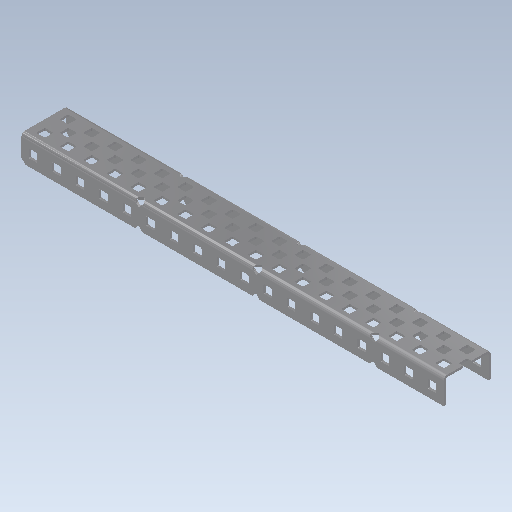
# Autodesk Inventor part: C-Channel 1x3x1x20 hole
Saved by Autodesk Inventor 2020.2 (Build 242310000, 310)
## iProperties
Created: 2012-03-22
Part Number: C-Channel 1x3x1x20 hole
Material: Aluminum 6061
Document SubType Name: Sheet Metal
Designer: Autodesk Inc.
Density: 2.7 g/cm^3
Sheet Metal Rule: Default
Vendor: VEX
Appearance: Aluminum - Polished
Category: Structure
Company: Autodesk Inc.
d52: 0.000 in
d53: 0.000 in
d54: 0.000 in
d55: 0.000 in
d56: 0.000 in
d57: 0.000 in
d58: 0.000 in
d59: 0.000 in
d60: 0.000 in
d61: 0.000 in
d62: 0.000 in
d63: 0.000 in
d64: 0.000 in
d65: 0.000 in
d66: 0.000 in
d67: 0.000 in
d68: 0.000 in
d69: 0.000 in
d70: 0.000 in
d71: 0.000 in
d72: 0.000 in
d73: 0.000 in
d74: 0.000 in
d75: 0.000 in
d76: 0.000 in
d77: 0.000 in
d78: 0.000 in
d79: 0.000 in
d80: 0.000 in
d81: 0.000 in
d82: 0.000 in
d83: 0.000 in
d84: 0.000 in
d85: 0.000 in
d86: 0.000 in
d87: 0.000 in
d88: 0.000 in
d89: 0.000 in
d90: 0.000 in
d91: 0.000 in
d92: 0.000 in
d93: 0.000 in
d94: 0.000 in
d95: 0.000 in
d96: 0.000 in
d97: 0.000 in
d98: 0.000 in
d99: 0.000 in
d100: 0.000 in
d101: 0.000 in
d102: 0.000 in
d103: 0.000 in
d104: 0.000 in
d105: 0.000 in
d106: 0.000 in
d107: 0.000 in
d108: 0.000 in
d109: 0.000 in
d110: 0.000 in
d111: 0.000 in
d112: 0.000 in
d113: 0.000 in
d114: 0.000 in
d115: 0.000 in
d116: 0.000 in
d117: 0.000 in
d118: 0.000 in
d119: 0.000 in
d120: 0.000 in
d121: 0.000 in
d122: 0.000 in
d123: 0.000 in
d124: 0.000 in
d125: 0.000 in
d126: 0.000 in
d127: 0.000 in
d128: 0.000 in
d129: 0.000 in
d130: 0.000 in
d131: 0.000 in
d132: 0.000 in
d133: 0.000 in
d134: 0.000 in
d135: 0.000 in
d136: 0.000 in
d137: 0.000 in
d138: 0.000 in
d139: 0.000 in
d140: 0.000 in
d141: 0.000 in
d142: 0.000 in
d143: 0.000 in
d144: 0.000 in
d145: 0.000 in
d146: 0.000 in
d147: 0.000 in
d148: 0.000 in
d149: 0.000 in
d150: 0.000 in
d151: 0.000 in
d152: 0.000 in
d153: 0.000 in
d154: 0.000 in
d155: 0.000 in
d156: 0.000 in
d157: 0.000 in
d158: 0.000 in
d159: 0.000 in
d160: 0.000 in
d161: 0.000 in
d162: 0.000 in
d163: 0.000 in
d164: 0.000 in
d165: 0.000 in
d166: 0.000 in
d167: 0.000 in
d168: 0.000 in
d169: 0.000 in
d361: 0.000 in
d362: 0.000 in
d363: 0.000 in
d364: 0.000 in
d365: 0.000 in
d366: 0.000 in
d367: 0.000 in
d368: 0.000 in
d369: 0.000 in
d370: 0.000 in
d371: 0.000 in
d372: 0.000 in
d373: 0.000 in
d374: 0.000 in
d375: 0.000 in
d376: 0.000 in
d377: 0.000 in
d378: 0.000 in
d379: 0.000 in
d380: 0.000 in
d381: 0.000 in
d382: 0.000 in
d383: 0.000 in
d384: 0.000 in
d385: 0.000 in
d386: 0.000 in
d387: 0.000 in
d388: 0.000 in
d389: 0.000 in
d390: 0.000 in
d391: 0.000 in
d392: 0.000 in
d393: 0.000 in
d394: 0.000 in
d395: 0.000 in
d396: 0.000 in
d397: 0.000 in
d398: 0.000 in
d399: 0.000 in
d400: 0.000 in
d401: 0.000 in
d402: 0.000 in
d403: 0.000 in
d404: 0.000 in
d405: 0.000 in
d406: 0.000 in
d407: 0.000 in
d408: 0.000 in
d409: 0.000 in
d410: 0.000 in
d411: 0.000 in
d412: 0.000 in
d413: 0.000 in
d414: 0.000 in
d415: 0.000 in
d416: 0.000 in
d417: 0.000 in
d418: 0.000 in
d419: 0.000 in
d420: 0.000 in
d421: 0.000 in
d422: 0.000 in
d423: 0.000 in
d424: 0.000 in
d425: 0.000 in
d426: 0.000 in
d427: 0.000 in
d428: 0.000 in
d429: 0.000 in
d430: 0.000 in
d431: 0.000 in
d432: 0.000 in
d433: 0.000 in
d434: 0.000 in
d435: 0.000 in
d436: 0.000 in
d437: 0.000 in
d438: 0.000 in
d439: 0.000 in
d440: 0.000 in
Author: Autodesk Inc.
Autodesk Inventor part; units mm, degrees
ref_plane "YZ Plane" through (0, 0, 0) normal (1, 0, 0) x (0, 1, 0)
sketch "Sketch1" plane through (0, 0, 0) normal (0, 0, 1) x (1, 0, 0)
  line L0 (0.7045, 9.1059) -> (254.7045, 9.1059)
  line L1 (254.7045, 9.1059) -> (254.7045, 22.9743)
  line L2 (254.7045, 22.9743) -> (0.7045, 22.9743)
  line L3 (0.7045, 22.9743) -> (0.7045, 9.1059)
  point P0 (0, 0)
  dimension "d0" = 254
  dimension "d1" = 13.8684
  measures "d0" distance of L2.end L1.end
  measures "d1" distance of L0.end L1.end
extrude "Plate1" add sketch "Sketch1" along normal blind 1.1684
sketch "Sketch2" plane through (0.7045, 21.8059, 0) normal (0, 1, 0) x (-1, 0, 0)
  line L0 (-254, 0) -> (0, 0)
  line L1 (0, 0) -> (0, 25.4)
  line L2 (0, 25.4) -> (-254, 25.4)
  line L3 (-254, 25.4) -> (-254, 0)
  constraints: 4 end point, 4 other
edge flange "Flange1" height 24.2316 angle 90 thickness 1.1684 bend radius 0.8128 thickness toward (0, 1, 0) relief tear relief width 1.1684 relief depth 0.5842 edges at (127.7045, 22.9743, 1.1684) wall of the first edge with corners at (254.7045, 21.8059, 0) (0.7045, 21.8059, 0) (0.7045, 21.8059, 25.4) (254.7045, 21.8059, 25.4)
bend "Bend1"
corner "Corner1"
sketch "Sketch3" plane through (254.7045, 21.8059, 25.4) normal (1, 0, 0) x (0, 0, -1)
  line L0 (23.4188, 0) -> (23.4188, 1.1684) projected
  line L1 (23.4188, 1.1684) -> (0, 1.1684) projected
  line L2 (0, 0) -> (0, 1.1684) projected
  line L3 (0, 0) -> (23.4188, 0) projected
  line L4 (23.4188, 0) -> (23.4188, 1.1684) projected
  arc A0 (24.2316, -0.8128) -> (23.4188, 0) centre (23.4188, -0.8128) ccw projected
  line L5 (25.4, -0.8128) -> (24.2316, -0.8128) projected
  arc A1 (25.4, -0.8128) -> (23.4188, 1.1684) centre (23.4188, -0.8128) ccw projected
  line L6 (25.4, -0.8128) -> (24.2316, -0.8128) projected
  line L7 (24.2316, -0.8128) -> (24.2316, -12.7) projected
  line L8 (25.4, -12.7) -> (24.2316, -12.7) projected
  line L9 (25.4, -12.7) -> (25.4, -0.8128) projected
  point P0 (25.4, -21.8059)
  dimension "d13" = 0.8128
  dimension "d14" = 1.9812
  measures "d13" radius of A0
  measures "d14" radius of A1
sketch "Sketch4" plane through (0.7045, 22.9743, 25.4) normal (0, 1, 0) x (1, 0, 0)
  line L0 (254, 23.4188) -> (254, 0) projected
  line L1 (249.4534, 4.0386) -> (245.8466, 4.0386)
  line L2 (245.3386, 4.5466) -> (245.3386, 8.1534)
  line L3 (245.8466, 8.6614) -> (249.4534, 8.6614)
  line L4 (249.9614, 8.1534) -> (249.9614, 4.5466)
  arc A0 (249.4534, 4.0386) -> (249.9614, 4.5466) centre (249.4534, 4.5466) ccw
  arc A1 (245.3386, 4.5466) -> (245.8466, 4.0386) centre (245.8466, 4.5466) ccw
  arc A2 (245.8466, 8.6614) -> (245.3386, 8.1534) centre (245.8466, 8.1534) ccw
  arc A3 (249.9614, 8.1534) -> (249.4534, 8.6614) centre (249.4534, 8.1534) ccw
  line L5 (254, 23.4188) -> (0, 23.4188) projected
  point P0 (-0.7045, 25.4)
  point P1 (249.9614, 4.0386)
  point P2 (245.3386, 8.6614)
  point P3 (245.3386, 4.0386)
  dimension "d15" = 4.6228
  dimension "d16" = 4.6228
  dimension "d18" = 4.0386
  dimension "d19" = 0.508
  dimension "d326" = 14.7574
  constraints: 8 end point, 8 point on circle, 8 tangent, 6 point on line, 4 centre point, 3 equal radius, 2 parallel, 1 horizontal, 1 perpendicular
  measures "d15" distance of point (249.961, 4.039) point (245.339, 4.039)
  measures "d16" distance of point (245.339, 4.039) point (245.339, 8.661)
  measures "d18" distance between parallel lines of L4 L0
  measures "d19" radius of A0
  measures "d326" distance between parallel lines of L3 L5
extrude "Cut1" cut sketch "Sketch4" against normal blind 1.1684
pattern_linear "Rectangular Pattern1" count 20 spacing 12.7 along (-1, 0, 0) count 2 spacing 12.7 along (0, 0, -1) of "Cut1"
sketch "Sketch5" plane through (0.7045, 22.9743, 25.4) normal (0, 1, 0) x (1, 0, 0)
  line L0 (249.4534, 4.0386) -> (245.8466, 4.0386) projected
  line L1 (249.9614, 8.1534) -> (249.9614, 4.5466) projected
  line L2 (243.1034, 10.3886) -> (239.4966, 10.3886)
  line L3 (238.9886, 10.8966) -> (238.9886, 14.5034)
  line L4 (239.4966, 15.0114) -> (243.1034, 15.0114)
  line L5 (243.6114, 14.5034) -> (243.6114, 10.8966)
  arc A0 (243.1034, 10.3886) -> (243.6114, 10.8966) centre (243.1034, 10.8966) ccw
  arc A1 (238.9886, 10.8966) -> (239.4966, 10.3886) centre (239.4966, 10.8966) ccw
  arc A2 (239.4966, 15.0114) -> (238.9886, 14.5034) centre (239.4966, 14.5034) ccw
  arc A3 (243.6114, 14.5034) -> (243.1034, 15.0114) centre (243.1034, 14.5034) ccw
  point P0 (-0.7045, 25.4)
  point P1 (243.6114, 10.3886)
  point P2 (238.9886, 15.0114)
  point P3 (238.9886, 10.3886)
  point P4 (243.6114, 15.0114)
  dimension "d28" = 4.6228
  dimension "d29" = 4.6228
  dimension "d30" = 6.35
  dimension "d31" = 6.35
  dimension "d34" = 0.508
  constraints: 8 end point, 8 point on circle, 8 point on line, 8 tangent, 4 centre point, 3 equal radius, 2 parallel, 1 horizontal, 1 perpendicular
  measures "d28" distance of point (243.611, 10.389) point (238.989, 10.389)
  measures "d29" distance of point (238.989, 10.389) point (238.989, 15.011)
  measures "d30" distance between parallel lines of L5 L1
  measures "d31" distance between parallel lines of L2 L0
  measures "d34" radius of A0
extrude "Cut2" cut sketch "Sketch5" against normal blind 1.1684
pattern_linear "Rectangular Pattern2" count 19 spacing 12.7 along (-1, 0, 0) of "Cut2"
sketch "Sketch6" plane through (0.7045, 22.9743, 25.4) normal (0, 1, 0) x (1, 0, 0)
  circle A0 centre (6.35, 19.05) radius 2.3114
  line L0 (4.5466, 21.3614) -> (8.1534, 21.3614) projected
  line L1 (8.6614, 20.8534) -> (8.6614, 17.2466) projected
  point P0 (-0.7045, 25.4)
  constraints: 2 tangent, 1 centre point
surface extrude "ExtrusionSrf1" sketch "Sketch6" against normal up to surface (1.1684 mm away) shown no curves A0
pattern_linear "Rectangular Pattern3" count 20 spacing 12.7 along (1, 0, 0) count 2 spacing 12.7 along (0, 0, 1) of "ExtrusionSrf1"
sketch "Sketch7" plane through (0.7045, 22.9743, 25.4) normal (0, 1, 0) x (1, 0, 0)
  line L0 (10.8966, 15.0114) -> (14.5034, 15.0114) projected
  line L1 (15.0114, 14.5034) -> (15.0114, 10.8966) projected
  circle A0 centre (12.7, 12.7) radius 2.3114
  point P0 (-0.7045, 25.4)
  constraints: 2 tangent, 1 centre point
surface extrude "ExtrusionSrf401" sketch "Sketch7" against normal up to surface (1.1684 mm away) shown no curves A0
pattern_linear "Rectangular Pattern4" count 19 spacing 12.7 along (1, 0, 0) of "ExtrusionSrf401"
ref_plane "Work Plane1" through (127.7045, 20.9931, 1.9812) normal (0, 0.7071068, 0.7071068) x (1, 0, 0)
sketch "Sketch11" plane through (0.7045, 22.9743, 24.2316) normal (0, 0, 1) x (1, 0, 0)
  line L0 (254, 0) -> (0, 0)
  line L1 (0, 0) -> (0, -13.8684)
  line L2 (0, -13.8684) -> (254, -13.8684)
  line L3 (254, -13.8684) -> (254, 0)
  constraints: 4 end point, 4 other
edge flange "Flange2" height 13.8684 angle 90 thickness 1.1684 bend radius 0.8128 thickness toward (0, 0, 1) relief tear relief width 1.1684 relief depth 0.5842 edges at (127.7045, 21.8059, 25.4) wall of the first edge with corners at (254.7045, 22.9743, 24.2316) (0.7045, 22.9743, 24.2316) (0.7045, 9.1059, 24.2316) (254.7045, 9.1059, 24.2316)
bend "Bend2"
corner "Corner2"
chamfer "Corner Chamfer1" distance 2.286 angle 45 4 edges at (254.7045, 9.1059, 0.5842) (0.7045, 9.1059, 0.5842) (0.7045, 9.1059, 24.8158) (254.7045, 9.1059, 24.8158)
sketch "Sketch8" plane through (0.7045, 22.9743, 1.9812) normal (0, 1, 0) x (1, 0, 0)
  line L0 (65.3034, -13.0302) -> (61.6966, -13.0302) projected
  line L1 (0, -21.4376) -> (254, -21.4376) projected
  line L2 (254, -23.4188) -> (0, -23.4188) projected
  line L3 (67.3002, -22.4282) -> (57.9533, -22.4282) construction
  line L4 (63.5, -20.2692) -> (61.1558, -22.4282)
  line L5 (63.5, -20.2692) -> (65.8442, -22.4282)
  line L6 (65.8442, -22.4282) -> (63.5, -24.5872)
  line L7 (63.5, -24.5872) -> (61.1558, -22.4282)
  point P0 (-0.7045, 1.9812)
  point P1 (63.5, -13.0302)
  dimension "d330" = 1.9812
  dimension "d331" = 0.9906
  dimension "d333" = 1.1684
  dimension "d334" = 94.71
  constraints: 10 end point, 3 equal length, 2 point on line, 1 midpoint, 1 parallel, 1 vertical alignment
  measures "d330" distance between parallel lines of L2 L1
  measures "d331" distance between parallel lines of L1 L3
  measures "d333" distance from line of L4.start L1
  measures "d334" angle of L4 L5
cut across bends "Cut6" sketch "Sketch8" k factor 0.44
pattern_linear "Rectangular Pattern8" count 3 spacing 63.5 along (1, 0, 0) of "Cut6"
ref_plane "Work Plane2" through (2.9905, 9.1059, 12.7) normal (0, 0, 1) x (1, 0, 0)
mirror "Mirror3" about plane through (2.9905, 9.1059, 12.7) normal (0, 0, 1) of "Cut6", "Rectangular Pattern8"
sketch "Sketch12" plane through (0, 0, 0) normal (0, 0, -1) x (-1, 0, 0)
  line L0 (-2.9905, 9.1059) -> (-252.4185, 9.1059) projected
  line L1 (-193.2365, 9.1059) -> (-191.2045, 11.1379)
  line L2 (-191.2045, 11.1379) -> (-189.1725, 9.1059)
  point P0 (-191.2045, 19.9278)
  point P1 (0, 0)
  dimension "d340" = 90
  dimension "d341" = 4.064
  constraints: 4 end point, 2 point on line, 1 perpendicular, 1 vertical alignment
  measures "d340" angle of L2 L1
  measures "d341" distance of L2.end L1.start
extrude "Cut7" cut sketch "Sketch12" against normal blind 1.1684
pattern_linear "Rectangular Pattern9" count 3 spacing 63.5 along (-1, 0, 0) of "Cut7"
mirror "Mirror4" about plane through (2.9905, 9.1059, 12.7) normal (0, 0, 1) of "Cut7", "Rectangular Pattern9"
sketch "Sketch13" plane through (0, 0, 0) normal (0, 0, -1) x (-1, 0, 0)
  line L0 (-254.7045, 11.3919) -> (-254.7045, 20.9931) projected
  line L1 (-250.1579, 13.1191) -> (-246.5511, 13.1191)
  line L2 (-246.0431, 13.6271) -> (-246.0431, 17.2339)
  line L3 (-246.5511, 17.7419) -> (-250.1579, 17.7419)
  line L4 (-250.6659, 17.2339) -> (-250.6659, 13.6271)
  line L5 (-254.7045, 22.9743) -> (-192.4731, 22.9743) projected
  arc A0 (-250.6659, 13.6271) -> (-250.1579, 13.1191) centre (-250.1579, 13.6271) ccw
  arc A1 (-250.1579, 17.7419) -> (-250.6659, 17.2339) centre (-250.1579, 17.2339) ccw
  arc A2 (-246.0431, 17.2339) -> (-246.5511, 17.7419) centre (-246.5511, 17.2339) ccw
  arc A3 (-246.5511, 13.1191) -> (-246.0431, 13.6271) centre (-246.5511, 13.6271) ccw
  point P0 (0, 0)
  point P1 (-250.6659, 13.1191)
  point P2 (-250.6659, 17.7419)
  dimension "d347" = 5.2324
  dimension "d348" = 4.6228
  dimension "d349" = 0.508
  dimension "d350" = 4.0386
  constraints: 8 end point, 8 point on circle, 8 tangent, 4 centre point, 4 point on line, 3 equal radius, 2 parallel, 2 perpendicular, 1 horizontal
  measures "d347" distance between parallel lines of L3 L5
  measures "d348" distance of point (-250.666, 17.742) point (-250.666, 13.119)
  measures "d349" radius of A0
  measures "d350" distance between parallel lines of L4 L0
extrude "Cut8" cut sketch "Sketch13" against normal blind 1.1684
pattern_linear "Rectangular Pattern10" count 20 spacing 12.7 along (-1, 0, 0) of "Cut8"
sketch "Sketch14" plane through (0, 0, 0) normal (0, 0, -1) x (-1, 0, 0)
  line L0 (-246.5511, 13.1191) -> (-250.1579, 13.1191) projected
  line L1 (-250.1579, 17.7419) -> (-246.5511, 17.7419) projected
  line L2 (-246.0431, 17.2339) -> (-246.0431, 13.6271) projected
  circle A0 centre (-248.3545, 15.4305) radius 2.3114
  point P0 (0, 0)
  constraints: 3 tangent, 1 centre point
surface extrude "ExtrusionSrf479" sketch "Sketch14" against normal up to surface (1.1684 mm away) shown no curves A0
pattern_linear "Rectangular Pattern11" count 20 spacing 12.7 along (-1, 0, 0) of "ExtrusionSrf479"
mirror "Mirror6" about plane through (2.9905, 9.1059, 12.7) normal (0, 0, 1) of "Cut8", "Rectangular Pattern10", "ExtrusionSrf479", "Rectangular Pattern11"
sketch "Sketch15" plane through (254.7045, 11.3919, 25.4) normal (0, 0, 1) x (1, 0, 0)
  line L0 (-25.4, 22.6832) -> (-25.4, -29.3145)
  line L1 (-29.4386, 5.842) -> (-29.4386, 2.2352) projected
  line L2 (-21.3614, 2.2352) -> (-21.3614, 5.842) projected
  line L3 (-25.4, 15.1451) -> (0.2602, 15.1451)
  line L4 (0.2602, 15.1451) -> (0.2602, -10.3325)
  line L5 (0.2602, -10.3325) -> (-25.4, -10.3325)
  line L6 (-25.4, -10.3325) -> (-25.4, 15.1451)
  point P0 (-254.7045, -11.3919)
  point P1 (-25.4, -10.3325)
  dimension "d442" = 4.0386
  constraints: 10 end point, 2 parallel, 1 horizontal, 1 perpendicular, 1 point on line, 1 vertical
  measures "d442" distance between parallel lines of L0 L1
extrude "Extrusion1" cut sketch "Sketch15" against normal blind 25.4
equation "\"d16\" = d15"
equation "\"d20\" = Thickness"
equation "\"d29\" = d28"
equation "\"d31\" = d30"
equation "\"d32\" = Thickness"
equation "\"d3\" = BendReliefWidth"
equation "\"d4\" = BendReliefDepth"
equation "\"d5\" = MinimumRemnant"
equation "\"d6\" = BendRadius"
equation "\"d9\" = BendRadius"
equation "\"d10\" = CornerReliefSize"
equation "\"d11\" = GapSize"
equation "\"d12\" = JacobiRadiusSize"
equation "\"BendRadius\" = 0.695652 * Thickness"
equation "\"BendReliefWidth\" = Thickness"
equation "\"BendReliefDepth\" = 0.5 * Thickness"
equation "\"CornerReliefSize\" = 4 * Thickness"
equation "\"MinimumRemnant\" = 2 * Thickness"
equation "\"TransitionRadius\" = BendRadius"
equation "\"JacobiRadiusSize\" = BendRadius"
equation "\"GapSize\" = Thickness"
equation "\"d2\" = BendRadius"
equation "\"Thickness\" = 1.1684"
body "Solid1"
body "Srf1"
body "Srf2"
body "Srf3"
body "Srf4"
body "Srf5"
body "Srf6"
body "Srf7"
body "Srf8"
body "Srf9"
body "Srf10"
body "Srf11"
body "Srf12"
body "Srf13"
body "Srf14"
body "Srf15"
body "Srf16"
body "Srf17"
body "Srf18"
body "Srf19"
body "Srf20"
body "Srf21"
body "Srf22"
body "Srf23"
body "Srf24"
body "Srf25"
body "Srf26"
body "Srf27"
body "Srf28"
body "Srf29"
body "Srf30"
body "Srf31"
body "Srf32"
body "Srf33"
body "Srf34"
body "Srf35"
body "Srf36"
body "Srf37"
body "Srf38"
body "Srf39"
body "Srf40"
body "Srf401"
body "Srf402"
body "Srf403"
body "Srf404"
body "Srf405"
body "Srf406"
body "Srf407"
body "Srf408"
body "Srf409"
body "Srf410"
body "Srf411"
body "Srf412"
body "Srf413"
body "Srf414"
body "Srf415"
body "Srf416"
body "Srf417"
body "Srf418"
body "Srf419"
body "Srf479"
body "Srf480"
body "Srf481"
body "Srf482"
body "Srf483"
body "Srf484"
body "Srf485"
body "Srf486"
body "Srf487"
body "Srf488"
body "Srf489"
body "Srf490"
body "Srf491"
body "Srf492"
body "Srf493"
body "Srf494"
body "Srf495"
body "Srf496"
body "Srf497"
body "Srf498"
body "Srf519"
body "Srf520"
body "Srf521"
body "Srf522"
body "Srf523"
body "Srf524"
body "Srf525"
body "Srf526"
body "Srf527"
body "Srf528"
body "Srf529"
body "Srf530"
body "Srf531"
body "Srf532"
body "Srf533"
body "Srf534"
body "Srf535"
body "Srf536"
body "Srf537"
body "Srf538"
